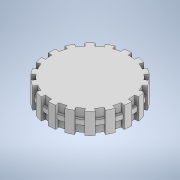
# Autodesk Inventor part: wheel
Saved by Autodesk Inventor 2022.1 (Build 261234000, 234)
## iProperties
Created: 2021-07-06
Part Number: wheel
Material: Generic
Document SubType Name: Modeling
Designer: dwbertol
Density: 1 g/cm^3
Appearance: Default
Sheet Metal Rule: Default_mm
Author: dwbertol
## iProperties of the stored document wheel_3DPrint.ipt
Created: 2021-07-16
Part Number: wheel_3DPrint
Material: Generic
Document SubType Name: Modeling
Designer: dwbertol
Density: 1 g/cm^3
Appearance: Default
Author: dwbertol
Autodesk Inventor part; units mm, degrees
ref_plane "YZ Plane" through (0, 0, 0) normal (1, 0, 0) x (0, 1, 0)
ref_plane "XZ Plane" through (0, 0, 0) normal (0, 1, 0) x (-1, 0, 0)
sketch "Sketch1" plane through (0, 0, 0) normal (0, 1, 0) x (-1, 0, 0)
  circle A0 centre (0, 0) radius 20.5
  circle A1 centre (0, 0) radius 1.55
  line L0 (-1, 1.1843) -> (-1, -1.1843)
  dimension "d0" = 41
  dimension "d3" = 3.1
  dimension "d12" = 1
  constraints: 2 centre point, 2 coincident, 2 end point, 2 point on circle, 1 vertical
  measures "d0" diameter of A0
  measures "d3" diameter of A1
  measures "d12" distance from line of point (0, 0) L0
extrude "Extrusion1" add sketch "Sketch1" along normal blind 8.5 contours A0 | L0 A1 picked at (-1.0868, -0.3007)
sketch "Sketch2" plane through (0, 0, 0) normal (0, -1, 0) x (1, 0, 0)
  arc A0 (1, 1.1843) -> (1, -1.1843) centre (0, 0) ccw projected
  circle A1 centre (0, 0) radius 20.5 projected
  line L0 (0, 17) -> (0, 15.5)
  line L1 (-2.952, 16.7417) -> (-2.6915, 15.2645)
  line L2 (-5.8143, 15.9748) -> (-5.3013, 14.5652)
  line L3 (-8.5, 14.7224) -> (-7.75, 13.4234)
  line L4 (-10.9274, 13.0228) -> (-9.9632, 11.8737)
  line L5 (-13.0228, 10.9274) -> (-11.8737, 9.9632)
  line L6 (-14.7224, 8.5) -> (-13.4234, 7.75)
  line L7 (-15.9748, 5.8143) -> (-14.5652, 5.3013)
  line L8 (-16.7417, 2.952) -> (-15.2645, 2.6915)
  line L9 (-17, 0) -> (-15.5, 0)
  line L10 (-16.7417, -2.952) -> (-15.2645, -2.6915)
  line L11 (-15.9748, -5.8143) -> (-14.5652, -5.3013)
  line L12 (-14.7224, -8.5) -> (-13.4234, -7.75)
  line L13 (-13.0228, -10.9274) -> (-11.8737, -9.9632)
  line L14 (-10.9274, -13.0228) -> (-9.9632, -11.8737)
  line L15 (-8.5, -14.7224) -> (-7.75, -13.4234)
  line L16 (-5.8143, -15.9748) -> (-5.3013, -14.5652)
  line L17 (-2.952, -16.7417) -> (-2.6915, -15.2645)
  line L18 (0, -17) -> (0, -15.5)
  line L19 (2.952, -16.7417) -> (2.6915, -15.2645)
  line L20 (5.8143, -15.9748) -> (5.3013, -14.5652)
  line L21 (8.5, -14.7224) -> (7.75, -13.4234)
  line L22 (10.9274, -13.0228) -> (9.9632, -11.8737)
  line L23 (13.0228, -10.9274) -> (11.8737, -9.9632)
  line L24 (14.7224, -8.5) -> (13.4234, -7.75)
  line L25 (15.9748, -5.8143) -> (14.5652, -5.3013)
  line L26 (16.7417, -2.952) -> (15.2645, -2.6915)
  line L27 (17, 0) -> (15.5, 0)
  line L28 (16.7417, 2.952) -> (15.2645, 2.6915)
  line L29 (15.9748, 5.8143) -> (14.5652, 5.3013)
  line L30 (14.7224, 8.5) -> (13.4234, 7.75)
  line L31 (13.0228, 10.9274) -> (11.8737, 9.9632)
  line L32 (10.9274, 13.0228) -> (9.9632, 11.8737)
  line L33 (8.5, 14.7224) -> (7.75, 13.4234)
  line L34 (5.8143, 15.9748) -> (5.3013, 14.5652)
  line L35 (2.952, 16.7417) -> (2.6915, 15.2645)
  arc A2 (5.3013, 14.5652) -> (2.6915, 15.2645) centre (0, 0) ccw
  arc A3 (8.5, 14.7224) -> (5.8143, 15.9748) centre (0, 0) ccw
  arc A4 (9.9632, 11.8737) -> (7.75, 13.4234) centre (0, 0) ccw
  arc A5 (13.0228, 10.9274) -> (10.9274, 13.0228) centre (0, 0) ccw
  arc A6 (13.4234, 7.75) -> (11.8737, 9.9632) centre (0, 0) ccw
  arc A7 (15.9748, 5.8143) -> (14.7224, 8.5) centre (0, 0) ccw
  arc A8 (15.2645, 2.6915) -> (14.5652, 5.3013) centre (0, 0) ccw
  arc A9 (17, 0) -> (16.7417, 2.952) centre (0, 0) ccw
  arc A10 (15.2645, -2.6915) -> (15.5, 0) centre (0, 0) ccw
  arc A11 (15.9748, -5.8143) -> (16.7417, -2.952) centre (0, 0) ccw
  arc A12 (13.4234, -7.75) -> (14.5652, -5.3013) centre (0, 0) ccw
  arc A13 (13.0228, -10.9274) -> (14.7224, -8.5) centre (0, 0) ccw
  arc A14 (9.9632, -11.8737) -> (11.8737, -9.9632) centre (0, 0) ccw
  arc A15 (8.5, -14.7224) -> (10.9274, -13.0228) centre (0, 0) ccw
  arc A16 (5.3013, -14.5652) -> (7.75, -13.4234) centre (0, 0) ccw
  arc A17 (2.952, -16.7417) -> (5.8143, -15.9748) centre (0, 0) ccw
  arc A18 (0, -15.5) -> (2.6915, -15.2645) centre (0, 0) ccw
  arc A19 (-2.952, -16.7417) -> (0, -17) centre (0, 0) ccw
  arc A20 (-5.3013, -14.5652) -> (-2.6915, -15.2645) centre (0, 0) ccw
  arc A21 (-8.5, -14.7224) -> (-5.8143, -15.9748) centre (0, 0) ccw
  arc A22 (-9.9632, -11.8737) -> (-7.75, -13.4234) centre (0, 0) ccw
  arc A23 (-13.0228, -10.9274) -> (-10.9274, -13.0228) centre (0, 0) ccw
  arc A24 (-13.4234, -7.75) -> (-11.8737, -9.9632) centre (0, 0) ccw
  arc A25 (-15.9748, -5.8143) -> (-14.7224, -8.5) centre (0, 0) ccw
  arc A26 (-15.2645, -2.6915) -> (-14.5652, -5.3013) centre (0, 0) ccw
  arc A27 (-17, 0) -> (-16.7417, -2.952) centre (0, 0) ccw
  arc A28 (-15.2645, 2.6915) -> (-15.5, 0) centre (0, 0) ccw
  arc A29 (-15.9748, 5.8143) -> (-16.7417, 2.952) centre (0, 0) ccw
  arc A30 (-13.4234, 7.75) -> (-14.5652, 5.3013) centre (0, 0) ccw
  arc A31 (-13.0228, 10.9274) -> (-14.7224, 8.5) centre (0, 0) ccw
  arc A32 (-9.9632, 11.8737) -> (-11.8737, 9.9632) centre (0, 0) ccw
  arc A33 (-8.5, 14.7224) -> (-10.9274, 13.0228) centre (0, 0) ccw
  arc A34 (0, 15.5) -> (-2.6915, 15.2645) centre (0, 0) ccw
  arc A35 (-5.3013, 14.5652) -> (-7.75, 13.4234) centre (0, 0) ccw
  arc A36 (2.952, 16.7417) -> (0, 17) centre (0, 0) ccw
  arc A37 (-2.952, 16.7417) -> (-5.8143, 15.9748) centre (0, 0) ccw
  line L36 (0, 17) -> (0, 15.5)
  arc A38 (0, 15.5) -> (-2.6915, 15.2645) centre (0, 0) ccw
  line L37 (-2.6915, 15.2645) -> (-2.952, 16.7417)
  arc A39 (-2.952, 16.7417) -> (-5.8143, 15.9748) centre (0, 0) ccw
  line L38 (-5.8143, 15.9748) -> (-5.3013, 14.5652)
  arc A40 (-5.3013, 14.5652) -> (-7.75, 13.4234) centre (0, 0) ccw
  line L39 (-7.75, 13.4234) -> (-8.5, 14.7224)
  arc A41 (-8.5, 14.7224) -> (-10.9274, 13.0228) centre (0, 0) ccw
  line L40 (-10.9274, 13.0228) -> (-9.9632, 11.8737)
  arc A42 (-9.9632, 11.8737) -> (-11.8737, 9.9632) centre (0, 0) ccw
  line L41 (-11.8737, 9.9632) -> (-13.0228, 10.9274)
  arc A43 (-13.0228, 10.9274) -> (-14.7224, 8.5) centre (0, 0) ccw
  line L42 (-14.7224, 8.5) -> (-13.4234, 7.75)
  arc A44 (-13.4234, 7.75) -> (-14.5652, 5.3013) centre (0, 0) ccw
  line L43 (-14.5652, 5.3013) -> (-15.9748, 5.8143)
  arc A45 (-15.9748, 5.8143) -> (-16.7417, 2.952) centre (0, 0) ccw
  line L44 (-16.7417, 2.952) -> (-15.2645, 2.6915)
  arc A46 (-15.2645, 2.6915) -> (-15.5, 0) centre (0, 0) ccw
  line L45 (-15.5, 0) -> (-17, 0)
  arc A47 (-17, 0) -> (-16.7417, -2.952) centre (0, 0) ccw
  line L46 (-16.7417, -2.952) -> (-15.2645, -2.6915)
  arc A48 (-15.2645, -2.6915) -> (-14.5652, -5.3013) centre (0, 0) ccw
  line L47 (-14.5652, -5.3013) -> (-15.9748, -5.8143)
  arc A49 (-15.9748, -5.8143) -> (-14.7224, -8.5) centre (0, 0) ccw
  line L48 (-14.7224, -8.5) -> (-13.4234, -7.75)
  arc A50 (-13.4234, -7.75) -> (-11.8737, -9.9632) centre (0, 0) ccw
  line L49 (-11.8737, -9.9632) -> (-13.0228, -10.9274)
  arc A51 (-13.0228, -10.9274) -> (-10.9274, -13.0228) centre (0, 0) ccw
  line L50 (-10.9274, -13.0228) -> (-9.9632, -11.8737)
  arc A52 (-9.9632, -11.8737) -> (-7.75, -13.4234) centre (0, 0) ccw
  line L51 (-7.75, -13.4234) -> (-8.5, -14.7224)
  arc A53 (-8.5, -14.7224) -> (-5.8143, -15.9748) centre (0, 0) ccw
  line L52 (-5.8143, -15.9748) -> (-5.3013, -14.5652)
  arc A54 (-5.3013, -14.5652) -> (-2.6915, -15.2645) centre (0, 0) ccw
  line L53 (-2.6915, -15.2645) -> (-2.952, -16.7417)
  arc A55 (-2.952, -16.7417) -> (0, -17) centre (0, 0) ccw
  line L54 (0, -17) -> (0, -15.5)
  arc A56 (0, -15.5) -> (2.6915, -15.2645) centre (0, 0) ccw
  line L55 (2.6915, -15.2645) -> (2.952, -16.7417)
  arc A57 (2.952, -16.7417) -> (5.8143, -15.9748) centre (0, 0) ccw
  line L56 (5.8143, -15.9748) -> (5.3013, -14.5652)
  arc A58 (5.3013, -14.5652) -> (7.75, -13.4234) centre (0, 0) ccw
  line L57 (7.75, -13.4234) -> (8.5, -14.7224)
  arc A59 (8.5, -14.7224) -> (10.9274, -13.0228) centre (0, 0) ccw
  line L58 (10.9274, -13.0228) -> (9.9632, -11.8737)
  arc A60 (9.9632, -11.8737) -> (11.8737, -9.9632) centre (0, 0) ccw
  line L59 (11.8737, -9.9632) -> (13.0228, -10.9274)
  arc A61 (13.0228, -10.9274) -> (14.7224, -8.5) centre (0, 0) ccw
  line L60 (14.7224, -8.5) -> (13.4234, -7.75)
  arc A62 (13.4234, -7.75) -> (14.5652, -5.3013) centre (0, 0) ccw
  line L61 (14.5652, -5.3013) -> (15.9748, -5.8143)
  arc A63 (15.9748, -5.8143) -> (16.7417, -2.952) centre (0, 0) ccw
  line L62 (16.7417, -2.952) -> (15.2645, -2.6915)
  arc A64 (15.2645, -2.6915) -> (15.5, 0) centre (0, 0) ccw
  line L63 (15.5, 0) -> (17, 0)
  arc A65 (17, 0) -> (16.7417, 2.952) centre (0, 0) ccw
  line L64 (16.7417, 2.952) -> (15.2645, 2.6915)
  arc A66 (15.2645, 2.6915) -> (14.5652, 5.3013) centre (0, 0) ccw
  line L65 (14.5652, 5.3013) -> (15.9748, 5.8143)
  arc A67 (15.9748, 5.8143) -> (14.7224, 8.5) centre (0, 0) ccw
  line L66 (14.7224, 8.5) -> (13.4234, 7.75)
  arc A68 (13.4234, 7.75) -> (11.8737, 9.9632) centre (0, 0) ccw
  line L67 (11.8737, 9.9632) -> (13.0228, 10.9274)
  arc A69 (13.0228, 10.9274) -> (10.9274, 13.0228) centre (0, 0) ccw
  line L68 (10.9274, 13.0228) -> (9.9632, 11.8737)
  arc A70 (9.9632, 11.8737) -> (7.75, 13.4234) centre (0, 0) ccw
  line L69 (7.75, 13.4234) -> (8.5, 14.7224)
  arc A71 (8.5, 14.7224) -> (5.8143, 15.9748) centre (0, 0) ccw
  line L70 (5.8143, 15.9748) -> (5.3013, 14.5652)
  arc A72 (5.3013, 14.5652) -> (2.6915, 15.2645) centre (0, 0) ccw
  line L71 (2.6915, 15.2645) -> (2.952, 16.7417)
  arc A73 (2.952, 16.7417) -> (0, 17) centre (0, 0) ccw
  line L72 (0, 0) -> (0, 2.9673) construction
  dimension "d15" = 0
  dimension "d8" = 360
  dimension "d13" = 3.5
  dimension "d14" = 5
  constraints: 146 end point, 72 collinear, 2 vertical, 327 other
extrude "Extrusion2" cut sketch "Sketch2" along normal through all both and the other way through all
sketch "Sketch3" plane through (0, 0, 0) normal (0, -1, 0) x (1, 0, 0)
  arc A0 (1, 1.1843) -> (1, -1.1843) centre (0, 0) ccw projected
  circle A1 centre (0, 0) radius 10
  circle A2 centre (0, 0) radius 11.2
  dimension "d16" = 20
  dimension "d17" = 1.2
  constraints: 2 centre point, 2 coincident
  measures "d16" diameter of A1
  measures "d17" radial gap between concentric circles of A2 A1
extrude "Extrusion3" add sketch "Sketch3" along normal blind 0.5
sketch "Sketch4" plane through (0, 8.5, 0) normal (0, 1, 0) x (1, 0, 0)
  arc A0 (1, 1.1843) -> (1, -1.1843) centre (0, 0) ccw projected
  line L0 (1, 1.1843) -> (1, -1.1843) projected
extrude "Extrusion4" add sketch "Sketch4" against normal blind 1
ref_plane "Work Plane1" through (0, 4.25, 0) normal (0, 1, 0) x (1, 0, 0)
sketch "Sketch5" plane through (0, 4.25, 0) normal (0, 1, 0) x (1, 0, 0)
  circle A0 centre (0, 0) radius 16.5
  arc A1 (5.8143, 15.9748) -> (2.952, 16.7417) centre (0, 0) ccw projected
  line L0 (0, -15.5) -> (0, -17) projected
  arc A2 (0, -17) -> (2.952, -16.7417) centre (0, 0) ccw projected
  line L1 (2.952, -16.7417) -> (2.6915, -15.2645) projected
  arc A3 (2.6915, -15.2645) -> (5.3013, -14.5652) centre (0, 0) ccw projected
  line L2 (5.3013, -14.5652) -> (5.8143, -15.9748) projected
  arc A4 (5.8143, -15.9748) -> (8.5, -14.7224) centre (0, 0) ccw projected
  line L3 (8.5, -14.7224) -> (7.75, -13.4234) projected
  arc A5 (7.75, -13.4234) -> (9.9632, -11.8737) centre (0, 0) ccw projected
  line L4 (9.9632, -11.8737) -> (10.9274, -13.0228) projected
  arc A6 (10.9274, -13.0228) -> (13.0228, -10.9274) centre (0, 0) ccw projected
  line L5 (13.0228, -10.9274) -> (11.8737, -9.9632) projected
  arc A7 (11.8737, -9.9632) -> (13.4234, -7.75) centre (0, 0) ccw projected
  line L6 (13.4234, -7.75) -> (14.7224, -8.5) projected
  arc A8 (14.7224, -8.5) -> (15.9748, -5.8143) centre (0, 0) ccw projected
  line L7 (15.9748, -5.8143) -> (14.5652, -5.3013) projected
  arc A9 (14.5652, -5.3013) -> (15.2645, -2.6915) centre (0, 0) ccw projected
  line L8 (15.2645, -2.6915) -> (16.7417, -2.952) projected
  arc A10 (16.7417, -2.952) -> (17, 0) centre (0, 0) ccw projected
  line L9 (17, 0) -> (15.5, 0) projected
  arc A11 (15.5, 0) -> (15.2645, 2.6915) centre (0, 0) ccw projected
  line L10 (15.2645, 2.6915) -> (16.7417, 2.952) projected
  arc A12 (16.7417, 2.952) -> (15.9748, 5.8143) centre (0, 0) ccw projected
  line L11 (15.9748, 5.8143) -> (14.5652, 5.3013) projected
  arc A13 (14.5652, 5.3013) -> (13.4234, 7.75) centre (0, 0) ccw projected
  line L12 (13.4234, 7.75) -> (14.7224, 8.5) projected
  arc A14 (14.7224, 8.5) -> (13.0228, 10.9274) centre (0, 0) ccw projected
  line L13 (13.0228, 10.9274) -> (11.8737, 9.9632) projected
  arc A15 (11.8737, 9.9632) -> (9.9632, 11.8737) centre (0, 0) ccw projected
  line L14 (9.9632, 11.8737) -> (10.9274, 13.0228) projected
  arc A16 (10.9274, 13.0228) -> (8.5, 14.7224) centre (0, 0) ccw projected
  line L15 (8.5, 14.7224) -> (7.75, 13.4234) projected
  arc A17 (7.75, 13.4234) -> (5.3013, 14.5652) centre (0, 0) ccw projected
  line L16 (5.3013, 14.5652) -> (5.8143, 15.9748) projected
  arc A18 (5.8143, 15.9748) -> (2.952, 16.7417) centre (0, 0) ccw projected
  line L17 (2.952, 16.7417) -> (2.6915, 15.2645) projected
  arc A19 (2.6915, 15.2645) -> (0, 15.5) centre (0, 0) ccw projected
  line L18 (0, 15.5) -> (0, 17) projected
  arc A20 (0, 17) -> (-2.952, 16.7417) centre (0, 0) ccw projected
  line L19 (-2.952, 16.7417) -> (-2.6915, 15.2645) projected
  arc A21 (-2.6915, 15.2645) -> (-5.3013, 14.5652) centre (0, 0) ccw projected
  line L20 (-5.3013, 14.5652) -> (-5.8143, 15.9748) projected
  arc A22 (-5.8143, 15.9748) -> (-8.5, 14.7224) centre (0, 0) ccw projected
  line L21 (-8.5, 14.7224) -> (-7.75, 13.4234) projected
  arc A23 (-7.75, 13.4234) -> (-9.9632, 11.8737) centre (0, 0) ccw projected
  line L22 (-9.9632, 11.8737) -> (-10.9274, 13.0228) projected
  arc A24 (-10.9274, 13.0228) -> (-13.0228, 10.9274) centre (0, 0) ccw projected
  line L23 (-13.0228, 10.9274) -> (-11.8737, 9.9632) projected
  arc A25 (-11.8737, 9.9632) -> (-13.4234, 7.75) centre (0, 0) ccw projected
  line L24 (-13.4234, 7.75) -> (-14.7224, 8.5) projected
  arc A26 (-14.7224, 8.5) -> (-15.9748, 5.8143) centre (0, 0) ccw projected
  line L25 (-15.9748, 5.8143) -> (-14.5652, 5.3013) projected
  arc A27 (-14.5652, 5.3013) -> (-15.2645, 2.6915) centre (0, 0) ccw projected
  line L26 (-15.2645, 2.6915) -> (-16.7417, 2.952) projected
  arc A28 (-16.7417, 2.952) -> (-17, 0) centre (0, 0) ccw projected
  line L27 (-17, 0) -> (-15.5, 0) projected
  arc A29 (-15.5, 0) -> (-15.2645, -2.6915) centre (0, 0) ccw projected
  line L28 (-15.2645, -2.6915) -> (-16.7417, -2.952) projected
  arc A30 (-16.7417, -2.952) -> (-15.9748, -5.8143) centre (0, 0) ccw projected
  line L29 (-15.9748, -5.8143) -> (-14.5652, -5.3013) projected
  arc A31 (-14.5652, -5.3013) -> (-13.4234, -7.75) centre (0, 0) ccw projected
  line L30 (-13.4234, -7.75) -> (-14.7224, -8.5) projected
  arc A32 (-14.7224, -8.5) -> (-13.0228, -10.9274) centre (0, 0) ccw projected
  line L31 (-13.0228, -10.9274) -> (-11.8737, -9.9632) projected
  arc A33 (-11.8737, -9.9632) -> (-9.9632, -11.8737) centre (0, 0) ccw projected
  line L32 (-9.9632, -11.8737) -> (-10.9274, -13.0228) projected
  arc A34 (-10.9274, -13.0228) -> (-8.5, -14.7224) centre (0, 0) ccw projected
  line L33 (-8.5, -14.7224) -> (-7.75, -13.4234) projected
  arc A35 (-7.75, -13.4234) -> (-5.3013, -14.5652) centre (0, 0) ccw projected
  line L34 (-5.3013, -14.5652) -> (-5.8143, -15.9748) projected
  arc A36 (-5.8143, -15.9748) -> (-2.952, -16.7417) centre (0, 0) ccw projected
  line L35 (-2.952, -16.7417) -> (-2.6915, -15.2645) projected
  arc A37 (-2.6915, -15.2645) -> (0, -15.5) centre (0, 0) ccw projected
  arc A38 (1, 1.1843) -> (1, -1.1843) centre (0, 0) ccw projected
  point P0 (2.8652, -16.2493)
  point P1 (5.6433, -15.5049)
  point P2 (8.25, -14.2894)
  point P3 (10.606, -12.6397)
  point P4 (12.6397, -10.606)
  point P5 (14.2894, -8.25)
  point P6 (15.5049, -5.6433)
  point P7 (16.2493, -2.8652)
  point P8 (16.5, 0)
  point P9 (16.2493, 2.8652)
  point P10 (15.5049, 5.6433)
  point P11 (14.2894, 8.25)
  point P12 (12.6397, 10.606)
  point P13 (10.606, 12.6397)
  point P14 (8.25, 14.2894)
  point P15 (5.6433, 15.5049)
  point P16 (2.8652, 16.2493)
  point P17 (0, 16.5)
  point P18 (-2.8652, 16.2493)
  point P19 (-5.6433, 15.5049)
  point P20 (-8.25, 14.2894)
  point P21 (-10.606, 12.6397)
  point P22 (-12.6397, 10.606)
  point P23 (-14.2894, 8.25)
  point P24 (-15.5049, 5.6433)
  point P25 (-16.2493, 2.8652)
  point P26 (-16.5, 0)
  point P27 (-16.2493, -2.8652)
  point P28 (-15.5049, -5.6433)
  point P29 (-14.2894, -8.25)
  point P30 (-12.6397, -10.606)
  point P31 (-10.606, -12.6397)
  point P32 (-8.25, -14.2894)
  point P33 (-5.6433, -15.5049)
  point P34 (-2.8652, -16.2493)
  point P35 (0, -16.5)
  dimension "d23" = 1
  constraints: 3 other
extrude "Extrusion5" add sketch "Sketch5" along normal mid plane 2 contours L9 A11 L10 A0 | A0 L7 A9 L8 | L11 A13 L12 A0 | A0 L5 A7 L6 | L13 A15 L14 A0 | A0 L3 A5 L4 | L15 A17 L16 A0 | A0 L1 A3 L2 | L17 A19 L18 A0 | A0 L35 A37 L0 | L19 A21 L20 A0 | A0 L33 A35 L34 | L21 A23 L22 A0 | A0 L31 A33 L32 | L23 A25 L24 A0 | A0 L29 A31 L30 | L25 A27 L26 A0 | A0 L27 A29 L28
equation "\"BendRadius\" = Thickness"
equation "\"BendReliefWidth\" = Thickness"
equation "\"BendReliefDepth\" = 0.5 * Thickness"
equation "\"CornerReliefSize\" = 4 * Thickness"
equation "\"MinimumRemnant\" = 2 * Thickness"
equation "\"TransitionRadius\" = BendRadius"
equation "\"JacobiRadiusSize\" = BendRadius"
equation "\"GapSize\" = Thickness"
equation "\"Thickness\" = 0.5"
body "Solid1"
